Autodesk Fusion 360 part; units mm, degrees
note: some values were not read from the file. Chosen so that the rebuilt part matches the saved one: which bodies a step acts on.
(part 2 of 2)
sketch "Sketch8" plane through (0, 0, 0) normal (0, 0, 1) x (1, 0, 0)
  circle A0 centre (54.0403, 93.6005) radius 13.3842
  circle A1 centre (54.0403, 93.6005) radius 7.5
  line L0 (60.7068, -2.8) -> (56.4767, -2.8)
  line L1 (56.4767, -2.8) -> (51.2198, -9.1772)
  line L2 (51.2198, -9.1772) -> (45.6537, -2.6601)
  line L3 (45.6537, -2.6601) -> (6.9138, -2.5879)
  line L4 (6.9138, -2.5879) -> (5.1366, -2.9784)
  line L5 (5.1366, -2.9784) -> (5.6805, -4.7148)
  line L6 (5.6805, -4.7148) -> (24.9109, -38.1665)
  line L7 (24.9109, -38.1665) -> (33.5576, -39.7691)
  line L8 (33.5576, -39.7691) -> (30.6632, -47.5103)
  line L9 (30.6632, -47.5103) -> (32.7783, -51.1737)
  line L10 (32.7783, -51.1737) -> (60.7068, -2.8)
  line L11 (27.9285, -53.9737) -> (25.8135, -50.3103)
  line L12 (25.8135, -50.3103) -> (17.6623, -48.9462)
  line L13 (17.6623, -48.9462) -> (20.5232, -40.8673)
  line L14 (20.5232, -40.8673) -> (1.2157, -7.2815)
  line L15 (1.2157, -7.2815) -> (-0.0111, -5.9377)
  line L16 (-0.0111, -5.9377) -> (-1.2429, -7.2769)
  line L17 (-1.2429, -7.2769) -> (-20.5977, -40.6567)
  line L18 (-20.5977, -40.6567) -> (-17.6623, -48.9462)
  line L19 (-17.6623, -48.9462) -> (-25.8135, -50.3103)
  line L20 (-25.8135, -50.3103) -> (-27.9285, -53.9737)
  line L21 (-27.9285, -53.9737) -> (27.9285, -53.9737)
  line L22 (-32.7783, -51.1737) -> (-30.6632, -47.5103)
  line L23 (-30.6632, -47.5103) -> (-33.5576, -39.7691)
  line L24 (-33.5576, -39.7691) -> (-25.1306, -38.2072)
  line L25 (-25.1306, -38.2072) -> (-5.6981, -4.6936)
  line L26 (-5.6981, -4.6936) -> (-5.1477, -2.9592)
  line L27 (-5.1477, -2.9592) -> (-6.9234, -2.5621)
  line L28 (-6.9234, -2.5621) -> (-45.5086, -2.4902)
  line L29 (-45.5086, -2.4902) -> (-51.2198, -9.1772)
  line L30 (-51.2198, -9.1772) -> (-56.4767, -2.8)
  line L31 (-56.4767, -2.8) -> (-60.7068, -2.8)
  line L32 (-60.7068, -2.8) -> (-32.7783, -51.1737)
  line L33 (-60.7068, 2.8) -> (-56.4767, 2.8)
  line L34 (-56.4767, 2.8) -> (-51.2198, 9.1772)
  line L35 (-51.2198, 9.1772) -> (-45.6537, 2.6601)
  line L36 (-45.6537, 2.6601) -> (-6.9138, 2.5879)
  line L37 (-6.9138, 2.5879) -> (-5.1366, 2.9784)
  line L38 (-5.1366, 2.9784) -> (-5.6805, 4.7148)
  line L39 (-5.6805, 4.7148) -> (-24.9109, 38.1665)
  line L40 (-24.9109, 38.1665) -> (-33.5576, 39.7691)
  line L41 (-33.5576, 39.7691) -> (-30.6632, 47.5103)
  line L42 (-30.6632, 47.5103) -> (-32.7783, 51.1737)
  line L43 (-32.7783, 51.1737) -> (-60.7068, 2.8)
  line L44 (66.4042, 2.8) -> (35.627, 56.1078)
  line L45 (35.627, 56.1078) -> (33.6443, 52.6737)
  line L46 (33.6443, 52.6737) -> (62.4389, 2.8)
  line L47 (62.4389, 2.8) -> (66.4042, 2.8)
  line L48 (62.4389, -2.8) -> (33.6443, -52.6737)
  line L49 (33.6443, -52.6737) -> (35.627, -56.1078)
  line L50 (35.627, -56.1078) -> (66.4042, -2.8)
  line L51 (66.4042, -2.8) -> (62.4389, -2.8)
  line L52 (28.7946, -55.4737) -> (-28.7946, -55.4737)
  line L53 (-28.7946, -55.4737) -> (-30.7773, -58.9078)
  line L54 (-30.7773, -58.9078) -> (30.7773, -58.9078)
  line L55 (30.7773, -58.9078) -> (28.7946, -55.4737)
  line L56 (-33.6443, -52.6737) -> (-62.4389, -2.8)
  line L57 (-62.4389, -2.8) -> (-66.4042, -2.8)
  line L58 (-66.4042, -2.8) -> (-35.627, -56.1078)
  line L59 (-35.627, -56.1078) -> (-33.6443, -52.6737)
  line L60 (-62.4389, 2.8) -> (-33.6443, 52.6737)
  line L61 (-33.6443, 52.6737) -> (-35.627, 56.1078)
  line L62 (-35.627, 56.1078) -> (-66.4042, 2.8)
  line L63 (-66.4042, 2.8) -> (-62.4389, 2.8)
  line L64 (-27.9285, 53.9737) -> (-25.8135, 50.3103)
  line L65 (-25.8135, 50.3103) -> (-17.6623, 48.9462)
  line L66 (-17.6623, 48.9462) -> (-20.5232, 40.8673)
  line L67 (-20.5232, 40.8673) -> (-1.2157, 7.2815)
  line L68 (-1.2157, 7.2815) -> (0.0111, 5.9377)
  line L69 (0.0111, 5.9377) -> (1.2429, 7.2769)
  line L70 (1.2429, 7.2769) -> (20.5977, 40.6567)
  line L71 (20.5977, 40.6567) -> (17.6623, 48.9462)
  line L72 (17.6623, 48.9462) -> (25.8135, 50.3103)
  line L73 (25.8135, 50.3103) -> (27.9285, 53.9737)
  line L74 (27.9285, 53.9737) -> (-27.9285, 53.9737)
  line L75 (-28.7946, 55.4737) -> (28.7946, 55.4737)
  line L76 (28.7946, 55.4737) -> (30.7773, 58.9078)
  line L77 (30.7773, 58.9078) -> (-30.7773, 58.9078)
  line L78 (-30.7773, 58.9078) -> (-28.7946, 55.4737)
  line L79 (-4, 0.0075) -> (-4.7989, 1.5168)
  line L80 (-4.7989, 1.5168) -> (-6.7523, 1.0876)
  line L81 (-6.7523, 1.0876) -> (-42.2523, 1.1537)
  line L82 (-42.2523, 1.1537) -> (-42.2563, -0.9962)
  line L83 (-42.2563, -0.9962) -> (-6.7563, -1.0624)
  line L84 (-6.7563, -1.0624) -> (-4.8046, -1.4989)
  line L85 (-4.8046, -1.4989) -> (-4, 0.0075)
  line L86 (-56.8409, 0) -> (-51.1995, -6.8437)
  line L87 (-51.1995, -6.8437) -> (-45.3544, 0)
  line L88 (-45.3544, 0) -> (-51.1995, 6.8437)
  line L89 (-51.1995, 6.8437) -> (-56.8409, 0)
  line L90 (-59.3235, 0) -> (-60.0719, 1.3)
  line L91 (-60.0719, 1.3) -> (-89.0719, 1.3)
  line L92 (-89.0719, 1.3) -> (-97.0393, 5.9)
  line L93 (-97.0393, 5.9) -> (-103.3231, 1.5)
  line L94 (-103.3231, 1.5) -> (-103.3231, -1.5)
  line L95 (-103.3231, -1.5) -> (-97.0393, -5.9)
  line L96 (-97.0393, -5.9) -> (-89.0719, -1.3)
  line L97 (-89.0719, -1.3) -> (-60.0719, -1.3)
  line L98 (-60.0719, -1.3) -> (-59.3235, 0)
  line L99 (-1.9935, 3.4678) -> (-1.0859, 4.9144)
  line L100 (-1.0859, 4.9144) -> (-2.4343, 6.3915)
  line L101 (-2.4343, 6.3915) -> (-20.127, 37.1684)
  line L102 (-20.127, 37.1684) -> (-21.9909, 36.0969)
  line L103 (-21.9909, 36.0969) -> (-4.2982, 5.32)
  line L104 (-4.2982, 5.32) -> (-3.7004, 3.4114)
  line L105 (-3.7004, 3.4114) -> (-1.9935, 3.4678)
  line L106 (-28.4205, 49.2257) -> (-31.5265, 40.9182)
  line L107 (-31.5265, 40.9182) -> (-22.6772, 39.2781)
  line L108 (-22.6772, 39.2781) -> (-19.673, 47.7619)
  line L109 (-19.673, 47.7619) -> (-28.4205, 49.2257)
  line L110 (-29.6618, 51.3757) -> (-28.9101, 52.6738)
  line L111 (-28.9101, 52.6738) -> (-43.4101, 77.7885)
  line L112 (-43.4101, 77.7885) -> (-43.4101, 86.9885)
  line L113 (-43.4101, 86.9885) -> (-50.3625, 90.2305)
  line L114 (-50.3625, 90.2305) -> (-52.9606, 88.7305)
  line L115 (-52.9606, 88.7305) -> (-53.6292, 81.0885)
  line L116 (-53.6292, 81.0885) -> (-45.6618, 76.4885)
  line L117 (-45.6618, 76.4885) -> (-31.1618, 51.3738)
  line L118 (-31.1618, 51.3738) -> (-29.6618, 51.3757)
  line L119 (2.0065, 3.4604) -> (3.7131, 3.3976)
  line L120 (3.7131, 3.3976) -> (4.318, 5.3039)
  line L121 (4.318, 5.3039) -> (22.1253, 36.0147)
  line L122 (22.1253, 36.0147) -> (20.2654, 37.0931)
  line L123 (20.2654, 37.0931) -> (2.4581, 6.3824)
  line L124 (2.4581, 6.3824) -> (1.1042, 4.9103)
  line L125 (1.1042, 4.9103) -> (2.0065, 3.4604)
  line L126 (28.4205, 49.2257) -> (19.673, 47.7619)
  line L127 (19.673, 47.7619) -> (22.6772, 39.2781)
  line L128 (22.6772, 39.2781) -> (31.5265, 40.9182)
  line L129 (31.5265, 40.9182) -> (28.4205, 49.2257)
  line L130 (29.6618, 51.3757) -> (31.1618, 51.3738)
  line L131 (31.1618, 51.3738) -> (45.6618, 76.4885)
  line L132 (45.6618, 76.4885) -> (53.6292, 81.0885)
  line L133 (53.6292, 81.0885) -> (52.9606, 88.7305)
  line L134 (52.9606, 88.7305) -> (50.3625, 90.2305)
  line L135 (50.3625, 90.2305) -> (43.4101, 86.9885)
  line L136 (43.4101, 86.9885) -> (43.4101, 77.7885)
  line L137 (43.4101, 77.7885) -> (28.9101, 52.6738)
  line L138 (28.9101, 52.6738) -> (29.6618, 51.3757)
  line L139 (59.3235, 0) -> (60.0719, -1.3)
  line L140 (60.0719, -1.3) -> (89.0719, -1.3)
  line L141 (89.0719, -1.3) -> (97.0393, -5.9)
  line L142 (97.0393, -5.9) -> (103.3231, -1.5)
  line L143 (103.3231, -1.5) -> (103.3231, 1.5)
  line L144 (103.3231, 1.5) -> (97.0393, 5.9)
  line L145 (97.0393, 5.9) -> (89.0719, 1.3)
  line L146 (89.0719, 1.3) -> (60.0719, 1.3)
  line L147 (60.0719, 1.3) -> (59.3235, 0)
  line L148 (56.8409, 0) -> (51.1995, 6.8437)
  line L149 (51.1995, 6.8437) -> (45.3544, 0)
  line L150 (45.3544, 0) -> (51.1995, -6.8437)
  line L151 (51.1995, -6.8437) -> (56.8409, 0)
  line L152 (4, -0.0075) -> (4.7989, -1.5168)
  line L153 (4.7989, -1.5168) -> (6.7523, -1.0876)
  line L154 (6.7523, -1.0876) -> (42.2523, -1.1537)
  line L155 (42.2523, -1.1537) -> (42.2563, 0.9962)
  line L156 (42.2563, 0.9962) -> (6.7563, 1.0624)
  line L157 (6.7563, 1.0624) -> (4.8046, 1.4989)
  line L158 (4.8046, 1.4989) -> (4, -0.0075)
  line L159 (29.6618, -51.3757) -> (28.9101, -52.6738)
  line L160 (28.9101, -52.6738) -> (43.4101, -77.7885)
  line L161 (43.4101, -77.7885) -> (43.4101, -86.9885)
  line L162 (43.4101, -86.9885) -> (50.3625, -90.2305)
  line L163 (50.3625, -90.2305) -> (52.9606, -88.7305)
  line L164 (52.9606, -88.7305) -> (53.6292, -81.0885)
  line L165 (53.6292, -81.0885) -> (45.6618, -76.4885)
  line L166 (45.6618, -76.4885) -> (31.1618, -51.3738)
  line L167 (31.1618, -51.3738) -> (29.6618, -51.3757)
  line L168 (28.4205, -49.2257) -> (31.5265, -40.9182)
  line L169 (31.5265, -40.9182) -> (22.6772, -39.2781)
  line L170 (22.6772, -39.2781) -> (19.673, -47.7619)
  line L171 (19.673, -47.7619) -> (28.4205, -49.2257)
  line L172 (1.9935, -3.4678) -> (1.0859, -4.9144)
  line L173 (1.0859, -4.9144) -> (2.4343, -6.3915)
  line L174 (2.4343, -6.3915) -> (20.127, -37.1684)
  line L175 (20.127, -37.1684) -> (21.9909, -36.0969)
  line L176 (21.9909, -36.0969) -> (4.2982, -5.32)
  line L177 (4.2982, -5.32) -> (3.7004, -3.4114)
  line L178 (3.7004, -3.4114) -> (1.9935, -3.4678)
  line L179 (-29.6618, -51.3757) -> (-31.1618, -51.3738)
  line L180 (-31.1618, -51.3738) -> (-45.6618, -76.4885)
  line L181 (-45.6618, -76.4885) -> (-53.6292, -81.0885)
  line L182 (-53.6292, -81.0885) -> (-52.9606, -88.7305)
  line L183 (-52.9606, -88.7305) -> (-50.3625, -90.2305)
  line L184 (-50.3625, -90.2305) -> (-43.4101, -86.9885)
  line L185 (-43.4101, -86.9885) -> (-43.4101, -77.7885)
  line L186 (-43.4101, -77.7885) -> (-28.9101, -52.6738)
  line L187 (-28.9101, -52.6738) -> (-29.6618, -51.3757)
  line L188 (-28.4205, -49.2257) -> (-19.673, -47.7619)
  line L189 (-19.673, -47.7619) -> (-22.6772, -39.2781)
  line L190 (-22.6772, -39.2781) -> (-31.5265, -40.9182)
  line L191 (-31.5265, -40.9182) -> (-28.4205, -49.2257)
  line L192 (-2.0065, -3.4604) -> (-3.7131, -3.3976)
  line L193 (-3.7131, -3.3976) -> (-4.318, -5.3039)
  line L194 (-4.318, -5.3039) -> (-22.1253, -36.0147)
  line L195 (-22.1253, -36.0147) -> (-20.2654, -37.0931)
  line L196 (-20.2654, -37.0931) -> (-2.4581, -6.3824)
  line L197 (-2.4581, -6.3824) -> (-1.1042, -4.9103)
  line L198 (-1.1042, -4.9103) -> (-2.0065, -3.4604)
  line L199 (-3.3169, 1.9233) -> (-2.3011, 0.0043)
  line L200 (-2.3011, 0.0043) -> (-3.324, -1.9109)
  line L201 (-3.324, -1.9109) -> (-1.1543, -1.9907)
  line L202 (-1.1543, -1.9907) -> (-0.0071, -3.8341)
  line L203 (-0.0071, -3.8341) -> (1.1469, -1.995)
  line L204 (1.1469, -1.995) -> (3.3169, -1.9233)
  line L205 (3.3169, -1.9233) -> (2.3011, -0.0043)
  line L206 (2.3011, -0.0043) -> (3.324, 1.9109)
  line L207 (3.324, 1.9109) -> (1.1543, 1.9907)
  line L208 (1.1543, 1.9907) -> (0.0071, 3.8341)
  line L209 (0.0071, 3.8341) -> (-1.1469, 1.995)
  line L210 (-1.1469, 1.995) -> (-3.3169, 1.9233)
  line L211 (60.7068, 2.8) -> (32.7783, 51.1737)
  line L212 (32.7783, 51.1737) -> (30.6632, 47.5103)
  line L213 (30.6632, 47.5103) -> (33.5576, 39.7691)
  line L214 (33.5576, 39.7691) -> (25.1306, 38.2072)
  line L215 (25.1306, 38.2072) -> (5.6981, 4.6936)
  line L216 (5.6981, 4.6936) -> (5.1477, 2.9592)
  line L217 (5.1477, 2.9592) -> (6.9234, 2.5621)
  line L218 (6.9234, 2.5621) -> (45.5086, 2.4902)
  line L219 (45.5086, 2.4902) -> (51.2198, 9.1772)
  line L220 (51.2198, 9.1772) -> (56.4767, 2.8)
  line L221 (56.4767, 2.8) -> (60.7068, 2.8)
  line L222 (68.1363, 2.8) -> (88.6699, 2.8)
  line L223 (88.6699, 2.8) -> (97.1169, 7.6768)
  line L224 (97.1169, 7.6768) -> (108.0805, 0)
  line L225 (108.0805, 0) -> (97.1169, -7.6768)
  line L226 (97.1169, -7.6768) -> (88.6699, -2.8)
  line L227 (88.6699, -2.8) -> (68.1363, -2.8)
  line L228 (68.1363, -2.8) -> (36.493, -57.6078)
  line L229 (36.493, -57.6078) -> (46.7598, -75.3904)
  line L230 (46.7598, -75.3904) -> (55.2068, -80.2673)
  line L231 (55.2068, -80.2673) -> (54.0403, -93.6005)
  line L232 (54.0403, -93.6005) -> (41.9101, -87.9441)
  line L233 (41.9101, -87.9441) -> (41.9101, -78.1904)
  line L234 (41.9101, -78.1904) -> (31.6433, -60.4078)
  line L235 (31.6433, -60.4078) -> (-31.6433, -60.4078)
  line L236 (-31.6433, -60.4078) -> (-41.9101, -78.1904)
  line L237 (-41.9101, -78.1904) -> (-41.9101, -87.9441)
  line L238 (-41.9101, -87.9441) -> (-54.0403, -93.6005)
  line L239 (-54.0403, -93.6005) -> (-55.2068, -80.2673)
  line L240 (-55.2068, -80.2673) -> (-46.7598, -75.3904)
  line L241 (-46.7598, -75.3904) -> (-36.493, -57.6078)
  line L242 (-36.493, -57.6078) -> (-68.1363, -2.8)
  line L243 (-68.1363, -2.8) -> (-88.6699, -2.8)
  line L244 (-88.6699, -2.8) -> (-97.1169, -7.6768)
  line L245 (-97.1169, -7.6768) -> (-108.0805, 0)
  line L246 (-108.0805, 0) -> (-97.1169, 7.6768)
  line L247 (-97.1169, 7.6768) -> (-88.6699, 2.8)
  line L248 (-88.6699, 2.8) -> (-68.1363, 2.8)
  line L249 (-68.1363, 2.8) -> (-36.493, 57.6078)
  line L250 (-36.493, 57.6078) -> (-46.7598, 75.3904)
  line L251 (-46.7598, 75.3904) -> (-55.2068, 80.2673)
  line L252 (-55.2068, 80.2673) -> (-54.0403, 93.6005)
  line L253 (-54.0403, 93.6005) -> (-41.9101, 87.9441)
  line L254 (-41.9101, 87.9441) -> (-41.9101, 78.1904)
  line L255 (-41.9101, 78.1904) -> (-31.6433, 60.4078)
  line L256 (-31.6433, 60.4078) -> (31.6433, 60.4078)
  line L257 (31.6433, 60.4078) -> (41.9101, 78.1904)
  line L258 (41.9101, 78.1904) -> (41.9101, 87.9441)
  line L259 (41.9101, 87.9441) -> (54.0403, 93.6005)
  line L260 (54.0403, 93.6005) -> (55.2068, 80.2673)
  line L261 (55.2068, 80.2673) -> (46.7598, 75.3904)
  line L262 (46.7598, 75.3904) -> (36.493, 57.6078)
  line L263 (36.493, 57.6078) -> (68.1363, 2.8)
  dimension "d457" = 15
  constraint concentric A0 A1
  constraint coincident A0 L260.end
  constraint coincident A0.centre A1.centre
  measures "d457" diameter of A1
extrude "Extrude8" add sketch "Sketch8" along normal up to surface (5 mm away) contours A0 A1 L259 L260 bodies 38
equation "d403 = 25 °"
equation "d404 = 124 °"
equation "d405 = 105.5 °"
equation "d416 = 30 °"
equation "d418 = 99 °"
equation "d419 = 80 °"
equation "d425 = 30 °"
equation "d430 = 60 °"
equation "d431 = 70 °"
